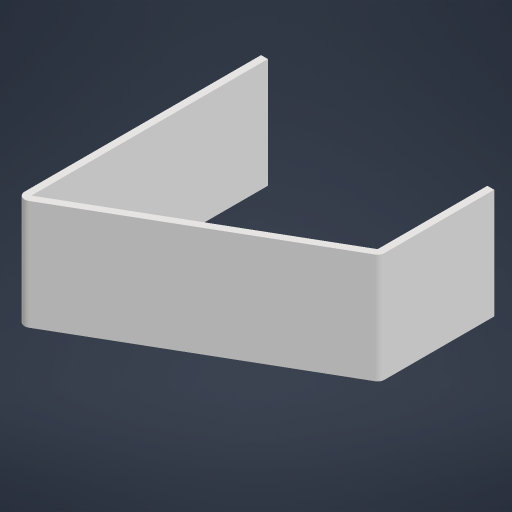
# Autodesk Inventor part: Part1
Saved by Autodesk Inventor 2023 (Build 270158000, 158)
## iProperties
Created: 2023-02-17
Part Number: Part1
Material: Generic
Document SubType Name: Modeling
Designer: Windows Macbook
Density: 1 g/cm^3
Appearance: Default
Author: Windows Macbook
Autodesk Inventor part; units mm, degrees
ref_plane "YZ Plane" through (0, 0, 0) normal (1, 0, 0) x (0, 1, 0)
ref_plane "XZ Plane" through (0, 0, 0) normal (0, 1, 0) x (-1, 0, 0)
ref_plane "XY Plane" through (0, 0, 0) normal (0, 0, 1) x (1, 0, 0)
sketch "Sketch1" plane through (0, 0, 0) normal (0, 1, 0) x (-1, 0, 0)
  line L0 (-1.5875, 0) -> (-1.5875, -25.4)
  line L1 (-1.5875, -25.4) -> (0, -25.4)
  line L2 (0, -25.4) -> (0, 0)
  line L3 (0, 0) -> (50.8, 29.3294)
  line L4 (50.8, 29.3294) -> (50.8, 0)
  line L5 (52.3875, 29.3294) -> (52.3875, -25.4076)
  line L6 (52.3875, -25.4076) -> (50.8, -25.4076)
  line L7 (50.8, -25.4076) -> (50.8, 29.3294)
  line L8 (-0.7937, 1.3748) -> (50.0062, 30.7042)
  arc A0 (52.3875, 29.3294) -> (50.0062, 30.7042) centre (50.8, 29.3294) ccw
  arc A1 (-0.7937, 1.3748) -> (-1.5875, 0) centre (0, 0) ccw
  dimension "d0" = 1.5875
  dimension "d1" = 25.4
  dimension "d5" = 1.5875
  dimension "d6" = 54.737
  dimension "d7" = 1.5875
  dimension "d8" = 1.5875
  constraints: 18 end point, 4 point on circle, 3 parallel, 2 centre point, 1 coincident, 1 point on line, 1 vertical
  measures "d0" distance of L1.end L0.end
  measures "d1" distance of L0.end L0.start
  measures "d5" distance of L5.end L6.end
  measures "d6" distance of L5.start L5.end
  measures "d7" distance of L3.end L8.end
  measures "d8" distance of L2.end L8.start
extrude "Extrusion1" add sketch "Sketch1" along normal blind 25.4
body "Solid1"
